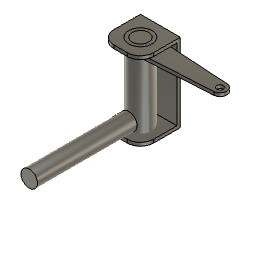
Main Assembly v35 (Autodesk Fusion 360 archive; units mm, degrees)
design "Spindle"
Autodesk Fusion 360 part; units mm, degrees
note: some values were not read from the file. Set by a fixed rule: the direction of a hole.
sketch "Sketch1" plane through (0, 0, 0) normal (0, 1, 0) x (1, 0, 0)
  line L0 (19.05, 34.29) -> (-19.05, 34.29)
  line L1 (-19.05, 34.29) -> (-19.05, -34.29)
  line L2 (-19.05, -34.29) -> (19.05, -34.29)
  line L3 (19.05, -34.29) -> (19.05, 34.29)
  line L4 (19.05, 34.29) -> (-19.05, -34.29) construction
  line L5 (-19.05, 34.29) -> (19.05, -34.29) construction
  dimension "d1" = 38.1
  dimension "d2" = 68.58
  constraint horizontal L0
  constraint perpendicular L0 L1
  constraint parallel L0 L2
  constraint parallel L1 L3
  constraint coincident L4 origin
  constraint coincident L5 origin
  measures "d1" distance of L1.end L2.end
  measures "d2" distance of L0.end L1.end
extrude "Extrude1" add sketch "Sketch1" along normal blind 3.175 makes body 1
box "BoxPrimitive1" add length 38.1 width 38.1 height 3.175 placed x (0, -1, 0) y (1, 0, 0) z (0, 0, 1) at (-19.05, 3.175, 34.29) separate body makes body 2
fillet "Fillet1" radius 12.7 2 edges at (19.05, -34.925, 35.8775) (-19.05, -34.925, 35.8775) on bodies 2
mirror "Mirror1" about plane through (0, 0, 0) normal (0, 0, 1) of bodies 2 makes body 3
combine "Combine1" operation add target body 2 tool bodies 1 3
copy_body "Body->Comp1" bodies 2 removing the originals makes body 4 in component "bracket"
sketch "Sketch1 (2)" plane through (0, 0, 0) normal (0, 0, 1) x (1, 0, 0) in component "axel"
  circle A0 centre (0, 0) radius 7.9375
  circle A1 centre (0, 0) radius 11.1125
  line L0 (0, 0) -> (0, -76.2) construction
  line L1 (-11.0908, -0.6945) -> (-6.3376, -76.5969)
  line L2 (11.0908, -0.6945) -> (6.3376, -76.5969)
  arc A2 (-6.3376, -76.5969) -> (6.3376, -76.5969) centre (0, -76.2) ccw
  dimension "d14" = 15.875
  dimension "d15" = 3.175
  dimension "d16" = 12.7
  dimension "d17" = 76.2
  constraint coincident A0.centre A1.centre
  constraint vertical L0
  constraint coincident L0.end A2.centre
  constraint coincident A1 L1.start
  constraint tangent L1 A2
  constraint tangent A1 L1
  constraint symmetric L0 L1.start L2.start
  constraint symmetric L0 L1.end L2.end
  measures "d14" diameter of A0
  measures "d16" diameter of A2
  measures "d17" distance of A0.centre L0.end
extrude "Extrude1'" add sketch "Sketch1 (2)" along normal blind 74.93 separate body contours A1 makes body 5 in component "axel"
extrude "Extrude2" add sketch "Sketch1 (2)" along normal blind 3.175 separate body contours A1 L1 L2 A2 makes body 6 in component "axel"
hole "Hole1" at (0, -76.2, 0) direction (0, 0, 1) diameter 6.35 end through all bodies 5 6 in component "axel"
ref_plane "WorkPlane1" through (-11.1125, 0, 31.4015) normal (-1, 0, 0) x (0, 1, 0) in component "axel"
cylinder "CylinderPrimitive1" add diameter 15.875 height 95.25 placed x (0, 0, 1) y (0, 1, 0) z (-1, 0, 0) at (-11.1125, 0, 11.0815) separate body makes body 7
copy_body "CutPasteBodies1" bodies 7 removing the originals makes body 8 in component "axel"
move_body "Move1" bodies 6 to x (1, 0, 0) y (0, 1, 0) z (0, 0, 1) at (0, 0, 68.326) in component "axel"
component "axel" placed x (0, 1, 0) y (-1, 0, 0) z (0, 0, 1) at (0, -15.875, -37.465)
component "bracket" placed x (1, 0, 0) y (0, 1, 0) z (0, 0, 1) at (0, 0, 0)
equation "thickness = 0.125 in"
equation "d7 = thickness"
equation "d14 = ( 5 / 8 ) * 1 in"
equation "d15 = thickness"
equation "d16 = ( 1 / 2 ) * 1 in"
equation "d20 = thickness"
named bodies: "bracket"

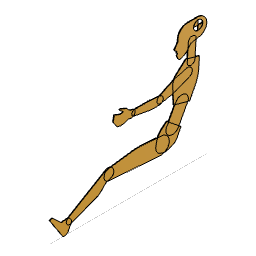
design "dummy"
Autodesk Fusion 360 part; units mm, degrees
sketch "Sketch1" plane through (0, 0, 0) normal (1, 0, 0) x (0, 0, -1)
  line L0 (377.4345, 358.9081) -> (405.7844, 402.0319)
  line L1 (405.7844, 402.0319) -> (405.7844, 416.5554)
  arc A0 (481.9229, 496.2148) -> (405.7844, 416.5554) centre (485.5252, 416.5554) ccw
  line L2 (481.9229, 496.2148) -> (566.8635, 496.2148)
  arc A1 (566.8635, 350.5394) -> (566.8635, 496.2148) centre (566.8635, 423.3771) ccw
  line L3 (566.8635, 350.5394) -> (509.6496, 339.5367)
  line L4 (509.6496, 339.5367) -> (484.1289, 305.0258)
  line L5 (449.829, 280.1877) -> (426.4866, 272.4668)
  line L6 (408.1258, 280.4895) -> (395.662, 307.8491)
  line L7 (395.662, 307.8491) -> (404.6842, 320.0495)
  line L8 (404.6842, 320.0495) -> (395.662, 325.0132)
  line L9 (395.662, 325.0132) -> (395.662, 342.1774)
  line L10 (395.662, 342.1774) -> (379.0932, 351.8425)
  line L11 (391.2001, 175.4409) -> (471.3746, 247.2021)
  line L12 (471.3746, 247.2021) -> (579.5678, 217.7571)
  line L13 (579.5678, 217.7571) -> (575.6146, 139.0874)
  line L14 (546.9286, 29.9053) -> (501.5044, -60.9431)
  line L15 (501.5044, -60.9431) -> (371.4651, -25.5527)
  line L16 (371.4651, -25.5527) -> (363.0601, 106.7151)
  line L17 (316.6173, -112.3007) -> (430.2886, -206.7985)
  line L18 (430.2886, -206.7985) -> (398.5225, -269.8892)
  line L19 (367.594, -299.7264) -> (340.9073, -311.9825)
  line L20 (262.8718, -310.581) -> (256.2942, -307.2692)
  line L21 (226.3165, -252.5216) -> (227.6439, -239.6069)
  line L22 (280.0646, -142.2074) -> (316.6173, -112.3007)
  line L23 (-157.8869, -295.0475) -> (262.5686, -326.8061)
  arc A2 (262.5686, -326.8061) -> (262.5686, -192.1775) centre (267.6531, -259.4918) ccw
  line L24 (262.5686, -192.1775) -> (122.4048, -181.5904)
  line L25 (34.8456, -184.029) -> (-157.8869, -209.4376)
  arc A3 (-157.8869, -209.4376) -> (-157.8869, -295.0475) centre (-152.2438, -252.2425) ccw
  line L26 (-208.2863, -226.6976) -> (-487.8996, -393.0848)
  arc A4 (-487.8996, -393.0848) -> (-460.2273, -439.5879) centre (-474.0634, -416.3364) ccw
  line L27 (-460.2273, -439.5879) -> (-253.7354, -362.3863)
  line L28 (-226.0749, -344.5947) -> (-176.5278, -295.0475)
  line L29 (-208.2863, -226.6976) -> (-179.2871, -209.4413)
  arc A5 (-142.0076, -285.3819) -> (-179.2871, -209.4413) centre (-157.5866, -245.9091) ccw
  line L30 (-142.0076, -285.3819) -> (-176.5278, -295.0475)
  line L31 (-634.9554, -338.5429) -> (-526.5621, -503.5493)
  line L32 (-526.5621, -503.5493) -> (-516.866, -503.5493)
  line L33 (-485.7312, -484.5374) -> (-469.2587, -452.4594)
  line L34 (-634.9554, -338.5429) -> (-626.4954, -332.9855)
  line L35 (-608.0708, -334.5141) -> (-541.0606, -396.5368)
  line L36 (-541.0606, -396.5368) -> (-497.315, -393.0848)
  arc A6 (-469.2587, -452.4594) -> (-497.315, -393.0848) centre (-494.5523, -428.0954) ccw
  line L37 (323.324, -136.2548) -> (388.9123, -14.0535)
  arc A7 (489.7112, -49.9544) -> (388.9123, -14.0535) centre (436.5908, -39.6436) ccw
  line L38 (489.7112, -49.9544) -> (409.3731, -199.637)
  arc A8 (323.324, -136.2548) -> (409.3731, -199.637) centre (361.8093, -174.1085) ccw
  line L39 (482.1167, 226.2068) -> (490.2849, 356.0025)
  arc A9 (553.2282, 356.0025) -> (490.2849, 356.0025) centre (521.7566, 354.022) ccw
  line L40 (553.2282, 356.0025) -> (544.3562, 215.0235)
  arc A10 (482.1167, 226.2068) -> (544.3562, 215.0235) centre (512.591, 217.0225) ccw
  line L41 (252.9029, 93.6494) -> (385.4603, 156.4761)
  line L42 (385.4603, 156.4761) -> (475.9031, 180.6402)
  arc A11 (495.257, 108.2013) -> (475.9031, 180.6402) centre (485.58, 144.4207) ccw
  line L43 (373.7234, 59.1292) -> (270.163, 38.4171)
  arc A12 (252.9029, 93.6494) -> (270.163, 38.4171) centre (264.457, 66.947) ccw
  line L44 (49.9244, 102.6246) -> (170.0545, 102.6246)
  line L45 (170.0545, 102.6246) -> (259.1165, 93.6494)
  arc A13 (256.044, 32.5174) -> (259.1165, 93.6494) centre (256.044, 63.1606) ccw
  line L46 (256.044, 32.5174) -> (187.418, 32.5174)
  line L47 (187.418, 32.5174) -> (49.234, 58.2688)
  arc A14 (49.9244, 102.6246) -> (49.234, 58.2688) centre (53.356, 80.3879) ccw
  line L48 (26.4507, 110.9095) -> (6.429, 122.6463)
  line L49 (6.429, 122.6463) -> (-7.379, 139.9064)
  line L50 (-7.379, 139.9064) -> (-66.9248, 165.6468)
  line L51 (-66.9248, 165.6468) -> (-69.701, 159.2244)
  line L52 (-69.701, 159.2244) -> (-37.1519, 131.2764)
  line L53 (-37.1519, 131.2764) -> (-61.9209, 124.7175)
  line L54 (-61.9209, 124.7175) -> (-111.6299, 145.2504)
  line L55 (-111.6299, 145.2504) -> (-119.9147, 97.7918)
  line L56 (-119.9147, 97.7918) -> (-86.7754, 49.4636)
  line L57 (-86.7754, 49.4636) -> (-53.2761, 43.6156)
  line L58 (-53.2761, 43.6156) -> (5.7386, 59.1292)
  line L59 (5.7386, 59.1292) -> (24.7321, 55.8135)
  arc A15 (24.7321, 55.8135) -> (26.4507, 110.9095) centre (29.5198, 83.239) ccw
  arc A16 (367.594, -299.7264) -> (398.5225, -269.8892) centre (340.4662, -240.6579) ccw
  arc A17 (262.8718, -310.581) -> (340.9073, -311.9825) centre (303.3459, -230.1953) ccw
  arc A18 (226.3165, -252.5216) -> (256.2942, -307.2692) centre (281.0284, -258.1446) ccw
  arc A19 (280.0646, -142.2074) -> (227.6439, -239.6069) centre (371.8841, -254.4312) ccw
  arc A20 (546.9286, 29.9053) -> (575.6146, 139.0874) centre (300.9611, 152.8891) ccw
  arc A21 (391.2001, 175.4409) -> (363.0601, 106.7151) centre (447.889, 112.1056) ccw
  line L60 (495.257, 108.2013) -> (373.7234, 59.1292)
  arc A22 (449.829, 280.1877) -> (484.1289, 305.0258) centre (427.8464, 346.6465) ccw
  arc A23 (408.1258, 280.4895) -> (426.4866, 272.4668) centre (421.7761, 286.7079) ccw
  arc A24 (377.4345, 358.9081) -> (379.0932, 351.8425) centre (381.6125, 356.1614) ccw
  arc A25 (-608.0708, -334.5141) -> (-626.4954, -332.9855) centre (-618.2598, -345.5225) ccw
  arc A26 (-516.866, -503.5493) -> (-485.7312, -484.5374) centre (-516.866, -468.5493) ccw
  arc A27 (122.4048, -181.5904) -> (34.8456, -184.029) centre (90.3942, -605.3832) ccw
  arc A28 (-253.7354, -362.3863) -> (-226.0749, -344.5947) centre (-280.8757, -289.7939) ccw
  circle A29 centre (569.6638, 438.2514) radius 34.9456
  circle A30 centre (569.6638, 438.2514) radius 37.6753
  line L61 (531.9886, 438.2514) -> (607.3391, 438.2514)
  line L62 (569.6638, 475.9267) -> (569.6638, 400.5761)
  dimension "d1" = 65
  dimension "d2" = 90
  dimension "d3" = 55
  dimension "d4" = 145
  dimension "d5" = 275
  dimension "d6" = 85
  dimension "d7" = 70
  dimension "d8" = 15
  dimension "d9" = 5
  dimension "d10" = 15
  dimension "d11" = 35
  dimension "d28" = 425
  dimension "d31" = 77.5
  dimension "d80" = 2.7296
  constraint vertical L1
  constraint tangent L1 A0
  constraint perpendicular L1 L2
  constraint tangent L2 A1
  constraint parallel L4 L7
  constraint vertical L9
  constraint parallel L12 L15
  constraint perpendicular L18 L20
  constraint tangent L23 A2
  constraint parallel L23 L24
  constraint tangent L25 A3
  constraint tangent L26 A4
  constraint parallel L26 L29
  constraint tangent L29 A5
  constraint horizontal L32
  constraint perpendicular L31 L34
  constraint tangent L36 A6
  constraint tangent L37 A7
  constraint parallel L37 L38
  constraint tangent L38 A8
  constraint tangent L39 A9
  constraint parallel L39 L40
  constraint tangent L40 A10
  constraint tangent L42 A11
  constraint tangent L43 A12
  constraint horizontal L44
  constraint tangent L45 A13
  constraint parallel L44 L46
  constraint tangent L47 A14
  constraint perpendicular L50 L51
  constraint perpendicular L55 L57
  constraint parallel L57 L59
  constraint tangent L59 A15
  constraint tangent L18 A16
  constraint tangent L19 A16
  constraint tangent L19 A17
  constraint tangent L20 A17
  constraint tangent L20 A18
  constraint tangent L21 A18
  constraint tangent L21 A19
  constraint tangent L22 A19
  constraint tangent L13 A20
  constraint tangent L14 A20
  constraint tangent L11 A21
  constraint tangent L16 A21
  constraint tangent L4 A22
  constraint tangent L5 A22
  constraint tangent L5 A23
  constraint tangent L6 A23
  constraint tangent L0 A24
  constraint tangent L10 A24
  constraint tangent A13 L46
  constraint tangent L34 A25
  constraint tangent L35 A25
  constraint tangent L32 A26
  constraint tangent L33 A26
  constraint tangent L24 A27
  constraint tangent L25 A27
  constraint tangent L27 A28
  constraint tangent L28 A28
  constraint coincident A30 L61.start
  constraint horizontal L61
  constraint vertical L62
  measures "d1" radius of A16
  measures "d2" radius of A17
  measures "d3" radius of A18
  measures "d4" radius of A19 L3.end
  measures "d5" radius of A20
  measures "d6" radius of A21
  measures "d7" radius of A22
  measures "d8" radius of A23
  measures "d9" radius of A24
  measures "d10" radius of A25
  measures "d11" radius of A26
  measures "d28" radius of A27
  measures "d31" radius of A28
extrude "Extrude1" add sketch "Sketch1" along normal blind 5 contours L0 L1 A0 L2 A1 L3 L4 L5 L6 L7 L8 L9 L10 L39 A9 L40 A22 A23 A24 | L3 L4 L39 A9 L40 | A29 L61 L62 | A29 A30 L61 L62 | A29 A30 L61 L62 | A29 L61 L62 | A29 L61 L62 | A29 A30 L61 L62 | A29 A30 L61 L62 | A29 L61 L62 makes body 1
extrude "Extrude2" add sketch "Sketch1" along normal blind 5 separate body contours L3 L4 L12 L39 L40 | L3 L4 L39 A9 L40 | L12 L39 L40 A10 makes body 2
extrude "Extrude3" add sketch "Sketch1" along normal blind 5 separate body contours L12 L39 L40 A10 | L11 L12 L13 L14 L15 L16 L37 A7 L38 L39 L40 A10 L41 L42 A11 L43 A20 A21 L60 | L16 L41 L42 A11 L43 A21 L60 | L15 L37 A7 L38 makes body 3
extrude "Extrude4" add sketch "Sketch1" along normal blind 5 separate body contours L16 L41 L43 L45 A13 A21 | L16 L41 L42 A11 L43 A21 L60 | L41 L43 A12 L45 A13 makes body 4
extrude "Extrude5" add sketch "Sketch1" along normal blind 5 separate body contours L41 L43 A12 L45 A13 | L41 L43 A12 L44 L45 A13 L46 L47 A14 A15 | A14 A15 makes body 5
extrude "Extrude6" add sketch "Sketch1" along normal blind 5 separate body contours A14 A15 | A14 L48 L49 L50 L51 L52 L53 L54 L55 L56 L57 L58 L59 A15 makes body 6
extrude "Extrude7" add sketch "Sketch1" along normal blind 5 separate body contours L15 L17 L37 L38 | L15 L37 A7 L38 | L17 L37 L38 A8 makes body 7
extrude "Extrude8" add sketch "Sketch1" along normal blind 5 separate body contours L17 L37 L38 A8 | L17 L18 L19 L22 A2 L24 L37 L38 A8 A16 A17 A19 | L20 L21 A2 L24 A17 A18 A19 makes body 8
extrude "Extrude9" add sketch "Sketch1" along normal blind 5 separate body contours L20 L21 L23 A2 L24 L25 A3 A5 L30 A17 A18 A19 A27 | L20 L21 A2 L24 A17 A18 A19 | L25 A3 A5 L30 makes body 9
extrude "Extrude10" add sketch "Sketch1" along normal blind 5 separate body contours L25 A3 A5 L30 | L25 A3 L26 A4 L27 L28 L29 A5 L30 A6 A28 | A4 A6 makes body 10
extrude "Extrude11" add sketch "Sketch1" along normal blind 5 separate body contours A4 A6 | A4 L31 L32 L33 L34 L35 L36 A6 A25 A26 makes body 11
copy_body "Body->Comp1" bodies 1 removing the originals makes body 12 in component "Head"
copy_body "Body->Comp2" bodies 2 removing the originals makes body 13 in component "neck"
copy_body "Body->Comp3" bodies 3 removing the originals makes body 14 in component "chest"
copy_body "Body->Comp4" bodies 4 removing the originals makes body 15 in component "upper arm"
copy_body "Body->Comp5" bodies 5 removing the originals makes body 16 in component "lower arm"
copy_body "Body->Comp6" bodies 6 removing the originals makes body 17 in component "hand"
copy_body "Body->Comp7" bodies 7 removing the originals makes body 18 in component "belly"
copy_body "Body->Comp8" bodies 8 removing the originals makes body 19 in component "pelvis"
copy_body "Body->Comp9" bodies 9 removing the originals makes body 20 in component "thigh"
copy_body "Body->Comp10" bodies 10 removing the originals makes body 21 in component "shin"
copy_body "Body->Comp11" bodies 11 removing the originals makes body 22 in component "foot"
extrude "Extrude1'" cut sketch "Sketch1" along normal blind 225 contours A29 L61 L62 | A29 A30 L61 L62 | A29 A30 L61 L62 | A29 A30 L61 L62 | A29 A30 L61 L62 | A29 L61 L62 picked at (577.7846, 460.024) picked at (546.4853, 436.5937) bodies 12 makes body 23 at (0, 387.8245, -483.7179) in component "Head"
component "dummy" placed x (1, 0, 0) y (0, 1, 0) z (0, 0, 1) at (0, 0, 0)
component "Head" placed x (1, 0, 0) y (0, 1, 0) z (0, 0, 1) at (0, 0, 0) in component "dummy"
component "neck" placed x (1, 0, 0) y (0, 1, 0) z (0, 0, 1) at (0, 0, 0) in component "dummy"
component "hand" placed x (1, 0, 0) y (0, 1, 0) z (0, 0, 1) at (0, 0, 0) in component "dummy"
component "lower arm" placed x (1, 0, 0) y (0, 1, 0) z (0, 0, 1) at (0, 0, 0) in component "dummy"
component "foot" placed x (1, 0, 0) y (0, 1, 0) z (0, 0, 1) at (0, 0, 0) in component "dummy"
component "chest" placed x (1, 0, 0) y (0, 1, 0) z (0, 0, 1) at (0, 0, 0) in component "dummy"
component "upper arm" placed x (1, 0, 0) y (0, 1, 0) z (0, 0, 1) at (0, 0, 0) in component "dummy"
component "shin" placed x (1, 0, 0) y (0, 1, 0) z (0, 0, 1) at (0, 0, 0) in component "dummy"
component "pelvis" placed x (1, 0, 0) y (0, 1, 0) z (0, 0, 1) at (0, 0, 0) in component "dummy"
component "belly" placed x (1, 0, 0) y (0, 1, 0) z (0, 0, 1) at (0, 0, 0) in component "dummy"
component "thigh" placed x (1, 0, 0) y (0, 1, 0) z (0, 0, 1) at (0, 0, 0) in component "dummy"
named bodies: "head", "neck", "chest", "upper arm", "lower arm", "hand", "Belly", "pelvis", "thigh", "shin", "foot", "head (1)"
